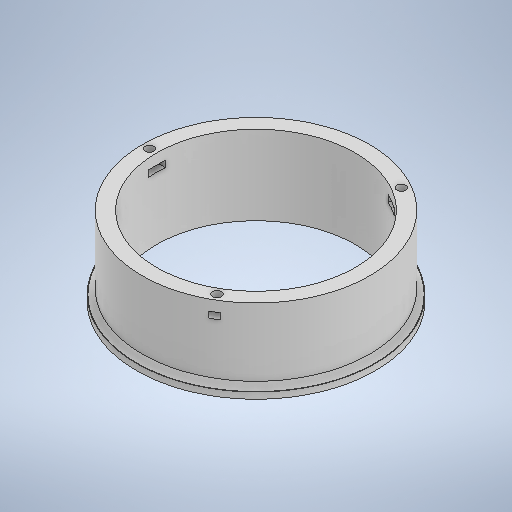
# Autodesk Inventor part: CenterCylinder_2
Saved by Autodesk Inventor 2025 (Build 290162000, 162)
## iProperties
Created: 2025-09-05
Part Number: CenterCylinder_2
Material: Generic
Document SubType Name: Modeling
Designer: mumin
Density: 1 g/cm^3
Appearance: Default
Author: mumin
Autodesk Inventor part; units mm, degrees
note: some values were not read from the file. Chosen so that the rebuilt part matches the saved one: direction of "Hole1".
ref_plane "YZ Plane" through (0, 0, 0) normal (1, 0, 0) x (0, 1, 0)
ref_plane "XZ Plane" through (0, 0, 0) normal (0, 1, 0) x (-1, 0, 0)
ref_plane "XY Plane" through (0, 0, 0) normal (0, 0, 1) x (1, 0, 0)
sketch "Sketch1" plane through (0, 0, 0) normal (0, 1, 0) x (-1, 0, 0)
  circle A0 centre (0, 0) radius 51
  circle A1 centre (0, 0) radius 47.55
  circle A2 centre (0, 0) radius 54.45
  dimension "d0" = 102
  dimension "d6" = 95.1
  dimension "d7" = 108.9
  constraints: 3 centre point, 2 coincident
  measures "d0" diameter of A0
  measures "d6" diameter of A1
  measures "d7" diameter of A2
extrude "Extrusion1" add sketch "Sketch1" along normal blind 30 contours A0 | A2
sketch "Sketch2" plane through (0, 30, 0) normal (0, 1, 0) x (1, 0, 0)
  line L0 (-51, 3.9837) -> (-47.55, 1.9919)
  line L1 (-47.55, 1.9919) -> (-47.55, -1.9919)
  line L2 (-47.55, -1.9919) -> (-51, -3.9837)
  line L3 (-51, -3.9837) -> (-54.45, -1.9919)
  line L4 (-54.45, -1.9919) -> (-54.45, 1.9919)
  line L5 (-54.45, 1.9919) -> (-51, 3.9837)
  circle A0 centre (0, 0) radius 54.45 projected
  circle A1 centre (0, 0) radius 47.55 projected
  line L6 (-51, -3.9837) -> (-47.2749, -3.9837)
  line L7 (-47.2749, -3.9837) -> (-47.2749, 3.9837)
  line L8 (-47.2749, 3.9837) -> (-51, 3.9837)
  line L9 (-51, 3.9837) -> (-51, -3.9837)
  point P0 (-51, 0)
  point P1 (-54.4128, 2.0134)
  point P2 (-54.4128, -2.0134)
  point P3 (-47.3828, -3.9837)
  point P4 (-47.55, 0)
  point P5 (-47.3828, 3.9837)
  constraints: 20 end point, 2 parallel, 2 tangent, 1 horizontal, 1 perpendicular, 13 other
extrude "Extrusion2" cut sketch "Sketch2" against normal blind 3 contours L8 A1 L1 L0 | L9 L3 A0 L5 | L0 L1 L2 L9 | L8 L7 L6 A1 | A1 L6 L7 L8 | L2 L1 A1 L6
pattern_circular "Circular Pattern1" count 3 over 360 about axis through (0, 0, 0) along (0, 1, 0) of "Extrusion2"
sketch "Sketch3" plane through (0, 30, 0) normal (0, 1, 0) x (1, 0, 0)
  circle A0 centre (0, 0) radius 47.55
  circle A1 centre (0, 0) radius 54.45
  constraints: 2 centre point, 2 coincident
extrude "Extrusion3" add sketch "Sketch3" along normal blind 5
sketch "Sketch4" plane through (0, 35, 0) normal (0, 1, 0) x (1, 0, 0)
  line L0 (-76.23, 0) -> (76.23, 0) projected
  point P0 (0, 0)
  point P1 (-51, 0)
  dimension "d22" = 51
  constraints: 1 point on line
  measures "d22" distance of point (0, 0) point (-51, 0)
hole "Hole1" at (-51, 35, 0) direction (0, -1, 0) diameter 4.2 depth 5
pattern_circular "Circular Pattern2" count 3 over 360 about axis through (0, 0, 0) along (0, 1, 0) of "Hole1"
sketch "Sketch5" plane through (0, 0, 0) normal (0, -1, 0) x (1, 0, 0)
  circle A0 centre (0, 0) radius 47.55
  circle A1 centre (0, 0) radius 57.192
  constraints: 2 centre point, 2 coincident
extrude "Extrusion4" add sketch "Sketch5" along normal blind 3
chamfer "Chamfer2" distance 2.5 angle 45 1 edges at (54.45, 0, 0)
body "Solid1"
